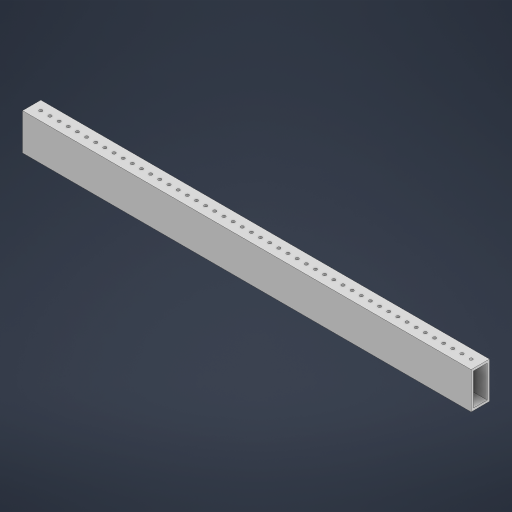
# Autodesk Inventor part: fram_support_24.5in
Saved by Autodesk Inventor 2023 (Build 270158000, 158)
## iProperties
Created: 2023-02-13
Part Number: fram_support_24.5in
Material: Generic
Document SubType Name: Modeling
Designer: bryce
Density: 1 g/cm^3
Appearance: Default
Author: bryce
Autodesk Inventor part; units mm, degrees
ref_plane "YZ Plane" through (0, 0, 0) normal (1, 0, 0) x (0, 1, 0)
ref_plane "XZ Plane" through (0, 0, 0) normal (0, 1, 0) x (-1, 0, 0)
ref_plane "XY Plane" through (0, 0, 0) normal (0, 0, 1) x (1, 0, 0)
sketch "Sketch1" plane through (0, 0, 0) normal (1, 0, 0) x (0, 1, 0)
  line L0 (0, 0) -> (50.8, 0)
  line L1 (50.8, 0) -> (50.8, -25.4)
  line L2 (50.8, -25.4) -> (0, -25.4)
  line L3 (0, -25.4) -> (0, 0)
  dimension "d0" = 50.8
  dimension "d1" = 25.4
  constraints: 8 end point, 2 parallel, 1 horizontal, 1 perpendicular
  measures "d0" distance of L1.end L2.end
  measures "d1" distance of L0.end L1.end
extrude "Extrusion1" add sketch "Sketch1" along normal blind 622.3
shell "Shell1" thickness 3.175 removed faces 2 at (0, 16.9333, -16.9333) at (622.3, 16.9333, -16.9333)
sketch "Sketch2" plane through (0, 50.8, 0) normal (0, 1, 0) x (1, 0, 0)
  line L0 (0, 22.225) -> (0, 3.175) projected
  line L1 (0, 12.7) -> (622.3, 12.7) construction
  line L2 (622.3, 3.175) -> (622.3, 22.225) projected
  circle A0 centre (12.7, 12.7) radius 2.0637
  line L3 (0, 25.4) -> (0, 0) projected
  dimension "d5" = 4.1275
  dimension "d6" = 12.7
  constraints: 3 midpoint, 2 end point, 1 centre point, 1 point on line
  measures "d5" diameter of A0
  measures "d6" distance of point (0, 12.7) A0.centre
hole "Hole1" at (12.7, 50.8, -12.7) direction (0, -1, 0) diameter 4.1275 end through all
pattern_linear "Rectangular Pattern1" count 48 spacing 12.7 along (1, 0, 0) of "Hole1"
body "Solid1"
